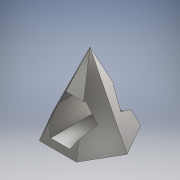
# Autodesk Inventor part: пирамида лаба
Saved by Autodesk Inventor 2018 (Build 220112000, 112)
## iProperties
Created: 2020-03-24
Part Number: пирамида лаба
Material: Сталь, высокопрочная, низколегированная
Document SubType Name: Modeling
Designer: 1
Mass: 110.935 g
Surface Area: 66.4661 cm^2
Volume: 14.1318 cm^3
Density: 7.85 g/cm^3
Appearance: Сталь — полированная
Author: 1
Autodesk Inventor part; units mm, degrees
ref_plane "YZ Plane" through (0, 0, 0) normal (1, 0, 0) x (0, 1, 0)
ref_plane "XZ Plane" through (0, 0, 0) normal (0, 1, 0) x (-1, 0, 0)
sketch "Эскиз1" plane through (0, 0, 0) normal (0, 0, 1) x (1, 0, 0)
  line L0 (-12.5, 21.6506) -> (12.5, 21.6506)
  line L1 (12.5, 21.6506) -> (25, 0)
  line L2 (25, 0) -> (12.5, -21.6506)
  line L3 (12.5, -21.6506) -> (-12.5, -21.6506)
  line L4 (-12.5, -21.6506) -> (-25, 0)
  line L5 (-25, 0) -> (-12.5, 21.6506)
  point P0 (0, 0)
  point P1 (0, 0)
  dimension "d0" = 50
  constraints: 12 end point, 1 coincident, 1 horizontal, 13 other
  measures "d0" distance of L1.end L4.end
ref_plane "РабПлоскость1" through (0, 0, 50) normal (0, 0, 1) x (1, 0, 0)
sketch "Эскиз2" plane through (0, 0, 50) normal (0, 0, 1) x (1, 0, 0)
  point P0 (0, 0)
  point P1 (0, 0)
loft "Лофт1" add profiles "Эскиз1" section 2 point at (0, 0, 50)
sketch "Эскиз3" plane through (0, 0, 0) normal (0, 1, 0) x (-1, 0, 0)
  line L0 (-6.5, 3.7417) -> (-13, 15)
  line L1 (-13, 15) -> (-6.5, 26.2583)
  line L2 (-6.5, 26.2583) -> (6.5, 26.2583)
  line L3 (6.5, 26.2583) -> (13, 15)
  line L4 (13, 15) -> (6.5, 3.7417)
  line L5 (6.5, 3.7417) -> (-6.5, 3.7417)
  line L6 (-12.5, 0) -> (12.5, 0) projected
  point P0 (0, 0)
  point P1 (0, 15)
  point P2 (0, 0)
  dimension "d6" = 26
  dimension "d7" = 15
  constraints: 12 end point, 1 horizontal, 1 midpoint, 1 vertical alignment, 13 other
  measures "d6" distance of L3.end L0.end
  measures "d7" distance of point (0, 0) point (0, 15)
extrude "Выдавливание1" cut sketch "Эскиз3" along normal through all both and the other way through all
